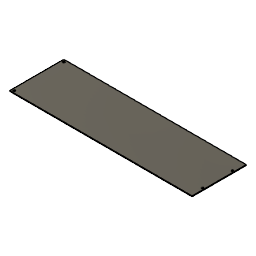
lid (Autodesk Fusion 360 design; units mm, degrees)
part number: 2026-05-27-13-07-37-797
Autodesk Fusion 360 part; units mm, degrees
sketch "Sketch1" plane through (0, 0, 0) normal (0, 0, 1) x (1, 0, 0)
  line L0 (0, 0) -> (458.394, 0)
  line L1 (458.394, 0) -> (458.394, 136.394)
  line L2 (458.394, 136.394) -> (0, 136.394)
  line L3 (0, 136.394) -> (0, 0)
  circle A0 centre (5.924, 130.475) radius 2.3
  circle A1 centre (5.924, 5.919) radius 2.3
  circle A2 centre (454.099, 30.516) radius 2.3
  circle A3 centre (454.099, 105.878) radius 2.3
  dimension "d1" = 136.394
  dimension "d2" = 458.394
  dimension "d3" = 4.6
  dimension "d4" = 5.919
  dimension "d5" = 5.924
  dimension "d6" = 4.6
  dimension "d7" = 5.919
  dimension "d8" = 5.924
  dimension "d9" = 4.6
  dimension "d10" = 4.295
  dimension "d11" = 30.516
  dimension "d12" = 4.6
  dimension "d13" = 30.516
  dimension "d14" = 4.295
  constraint horizontal L0
  constraint vertical L1
  constraint horizontal L2
  constraint vertical L3
  constraint coincident L0.start L3.end
  measures "d1" distance of L0.start L2.end
  measures "d2" distance of L0.start L0.end
  measures "d3" diameter of A0
  measures "d4" distance of L2 A0.centre
  measures "d5" distance of L3 A0.centre
  measures "d6" diameter of A1
  measures "d7" distance of L0 A1.centre
  measures "d8" distance of L3 A1.centre
  measures "d9" diameter of A2
  measures "d10" distance of L1 A2.centre
  measures "d11" distance of L0 A2.centre
  measures "d12" diameter of A3
  measures "d13" distance of L2 A3.centre
  measures "d14" distance of L1 A3.centre
extrude "Extrude1" add sketch "Sketch1" along normal blind 1.5
